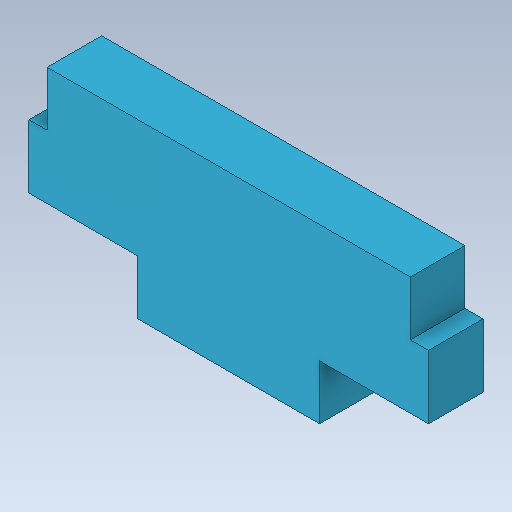
# Autodesk Inventor part: Celda sos deslizador
Saved by Autodesk Inventor 2020 (Build 240168000, 168)
## iProperties
Created: 2020-03-13
Part Number: Celda sos deslizador
Material: Genérico
Document SubType Name: Modeling
Designer: joser
Density: 1 g/cm^3
Appearance: Turquesa
Author: joser
Autodesk Inventor part; units mm, degrees
ref_plane "YZ Plane" through (0, 0, 0) normal (1, 0, 0) x (0, 1, 0)
ref_plane "XZ Plane" through (0, 0, 0) normal (0, 1, 0) x (-1, 0, 0)
ref_plane "XY Plane" through (0, 0, 0) normal (0, 0, 1) x (1, 0, 0)
sketch "Boceto1" plane through (0, 0, 0) normal (0, 0, 1) x (1, 0, 0)
  line L0 (22, 3.5) -> (22, 0)
  line L1 (0, 0) -> (0, 3.5)
  line L2 (1, 3.5) -> (1, 6.5)
  line L3 (1, 6.5) -> (21, 6.5)
  line L4 (21, 6.5) -> (21, 3.5)
  line L5 (0, 3.5) -> (1, 3.5)
  line L6 (21, 3.5) -> (22, 3.5)
  line L7 (6, 0) -> (6, -3)
  line L8 (6, -3) -> (16, -3)
  line L9 (16, -3) -> (16, 0)
  line L10 (22, 0) -> (16, 0)
  line L11 (6, 0) -> (0, 0)
  dimension "d5" = 20
  dimension "d6" = 1
  dimension "d7" = 3
  dimension "d9" = 22
  dimension "d11" = 10
  dimension "d12" = 6
  dimension "d13" = 3
  dimension "d14" = 3.5
  constraints: 24 end point, 7 perpendicular, 5 parallel, 2 collinear, 2 horizontal, 2 vertical, 1 coincident
  measures "d5" distance of L2.end L3.end
  measures "d6" distance between parallel lines of L1 L2
  measures "d7" distance between parallel lines of L5 L3
  measures "d9" distance between parallel lines of L1 L0
  measures "d11" distance of L7.end L8.end
  measures "d12" distance between parallel lines of L1 L7
  measures "d13" distance between parallel lines of L10 L8
  measures "d14" distance between parallel lines of L5 L11
extrude "Extrusión1" add sketch "Boceto1" along normal blind 3
